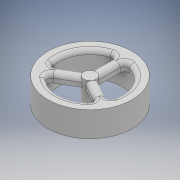
# Autodesk Inventor part: wheel
Saved by Autodesk Inventor 2018 (Build 220112000, 112)
## iProperties
Created: 2020-06-04
Part Number: wheel
Material: Generico
Document SubType Name: Modeling
Designer: Andrea Gotelli
Density: 1 g/cm^3
Appearance: Default
Author: Andrea Gotelli
Autodesk Inventor part; units mm, degrees
ref_plane "YZ Plane" through (0, 0, 0) normal (1, 0, 0) x (0, 1, 0)
ref_plane "XZ Plane" through (0, 0, 0) normal (0, 1, 0) x (-1, 0, 0)
ref_plane "XY Plane" through (0, 0, 0) normal (0, 0, 1) x (1, 0, 0)
sketch "Schizzo1" plane through (0, 0, 0) normal (0, 0, 1) x (1, 0, 0)
  circle A0 centre (0, 0) radius 50
  circle A1 centre (0, 0) radius 37.5
  circle A2 centre (0, 0) radius 7.5
  dimension "d0" = 100
  dimension "d1" = 75
  dimension "d2" = 15
  constraints: 3 centre point, 3 coincident
  measures "d0" diameter of A0
  measures "d1" diameter of A1
  measures "d2" diameter of A2
extrude "Estrusione1" add sketch "Schizzo1" along normal blind 30
sketch "Schizzo2" plane through (0, 0, 30) normal (0, 0, 1) x (1, 0, 0)
  line L0 (-5, 39.5) -> (-5, 4.5)
  line L1 (-5, 4.5) -> (5, 4.5)
  line L2 (5, 4.5) -> (5, 39.5)
  line L3 (5, 39.5) -> (-5, 39.5)
  line L4 (-5, 39.5) -> (5, 4.5) construction
  line L5 (-5, 4.5) -> (5, 39.5) construction
  line L6 (-31.708, -24.0801) -> (-1.3971, -6.5801)
  line L7 (-1.3971, -6.5801) -> (-6.3971, 2.0801)
  line L8 (-6.3971, 2.0801) -> (-36.708, -15.4199)
  line L9 (-36.708, -15.4199) -> (-31.708, -24.0801)
  line L10 (-31.708, -24.0801) -> (-6.3971, 2.0801) construction
  line L11 (-1.3971, -6.5801) -> (-36.708, -15.4199) construction
  line L12 (36.708, -15.4199) -> (6.3971, 2.0801)
  line L13 (6.3971, 2.0801) -> (1.3971, -6.5801)
  line L14 (1.3971, -6.5801) -> (31.708, -24.0801)
  line L15 (31.708, -24.0801) -> (36.708, -15.4199)
  line L16 (36.708, -15.4199) -> (1.3971, -6.5801) construction
  line L17 (6.3971, 2.0801) -> (31.708, -24.0801) construction
  point P0 (0, 0)
  point P1 (0, 22)
  point P2 (-19.0526, -11)
  point P3 (19.0526, -11)
  dimension "d5" = 22
  dimension "d6" = 0
  dimension "d7" = 10
  dimension "d8" = 35
  dimension "d11" = 360
  constraints: 36 end point, 6 midpoint, 2 parallel, 1 perpendicular, 1 vertical, 34 other
  measures "d5" distance of point (0, 0) point (0, 22)
  measures "d6" horizontal distance of point (0, 0) point (0, 22)
  measures "d7" distance of L0.end L1.end
  measures "d8" distance of L1.end L2.end
extrude "Estrusione2" add sketch "Schizzo2" against normal blind 10
fillet "Raccordo1" radius 5 6 edges at (-34.686, -14.2525, 25) (5, 37.1652, 25) (34.686, -14.2525, 25) (-5, 37.1652, 25) (29.686, -22.9127, 25) (-29.686, -22.9127, 25)
fillet "Raccordo2" radius 5 10 edges at (0, -37.5, 30) (13.3108, -13.4585, 30) (-13.3108, -13.4585, 30) (-5, 18.2567, 30) (-18.3108, -4.7982, 30) (-32.476, 18.75, 30) (30.3228, 22.0631, 30) (37.2918, -3.9458, 30) (18.3108, -4.7982, 30) (5, 18.2567, 30)
